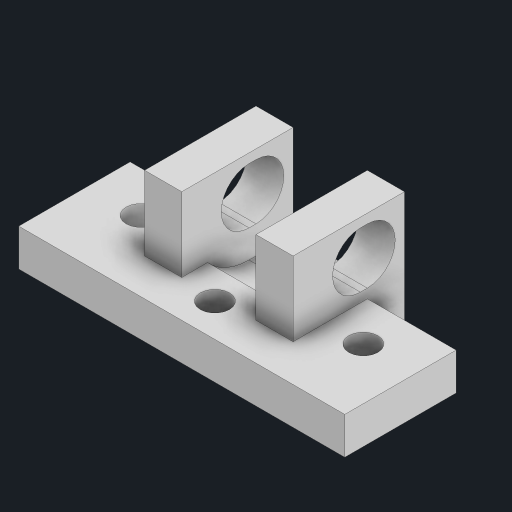
# Autodesk Inventor part: OUTK_005_LessUglyBracket
Saved by Autodesk Inventor 2024.2 (Build 282272000, 272)
## iProperties
Created: 2024-11-26
Part Number: OUTK_005_LessUglyBracket
Material: Generic
Document SubType Name: Modeling
Designer: Bryan
Density: 1 g/cm^3
Appearance: Default
Author: Bryan
Autodesk Inventor part; units mm, degrees
ref_plane "YZ Plane" through (0, 0, 0) normal (1, 0, 0) x (0, 1, 0)
ref_plane "XZ Plane" through (0, 0, 0) normal (0, 1, 0) x (-1, 0, 0)
ref_plane "XY Plane" through (0, 0, 0) normal (0, 0, 1) x (1, 0, 0)
sketch "Sketch1" plane through (0, 0, 0) normal (0, 1, 0) x (-1, 0, 0)
  circle A0 centre (0, 0) radius 2.4892
  circle A1 centre (19.05, -6.35) radius 2.4892
  circle A2 centre (-19.05, -6.35) radius 2.4892
  line L0 (21.5392, 2.4892) -> (-21.5392, 2.4892) construction
  line L1 (-21.5392, 2.4892) -> (-21.5392, -8.8392) construction
  line L2 (-21.5392, -8.8392) -> (21.5392, -8.8392) construction
  line L3 (21.5392, -8.8392) -> (21.5392, 2.4892) construction
  line L4 (27.8892, 5.6642) -> (-27.8892, 5.6642)
  line L5 (-27.8892, 5.6642) -> (-27.8892, -13.3858)
  line L6 (-27.8892, -13.3858) -> (27.8892, -13.3858)
  line L7 (27.8892, -13.3858) -> (27.8892, 5.6642)
  line L8 (12.7, -13.3858) -> (-12.7, -13.3858)
  line L9 (-12.7, -13.3858) -> (-12.7, -19.7358)
  line L10 (-12.7, -19.7358) -> (12.7, -19.7358)
  line L11 (12.7, -19.7358) -> (12.7, -13.3858)
  point P0 (21.5392, -3.175)
  point P1 (0, -19.7358)
  dimension "d0" = 4.9784
  dimension "d1" = 6.35
  dimension "d2" = 19.05
  dimension "d3" = 19.05
  dimension "d4" = 19.05
  dimension "d5" = 3.175
  dimension "d6" = 6.35
  dimension "d7" = 6.35
  dimension "d8" = 6.35
  dimension "d9" = 25.4
  constraints: 24 end point, 6 parallel, 4 tangent, 3 centre point, 3 horizontal, 3 perpendicular, 2 equal radius, 2 midpoint, 1 coincident, 1 horizontal alignment, 1 point on line, 1 vertical alignment
  measures "d0" diameter of A0
  measures "d1" vertical distance of A1.centre point (0, 0)
  measures "d2" horizontal distance of point (0, 0) A1.centre
  measures "d3" horizontal distance of A2.centre point (0, 0)
  measures "d4" distance of L5.end L4.end
  measures "d5" distance between parallel lines of L0 L4
  measures "d6" distance from line of point (21.539, -3.175) L7
  measures "d7" distance between parallel lines of L5 L1
  measures "d8" distance of L9.end L8.end
  measures "d9" distance of L9.end L10.end
extrude "Extrusion1" add sketch "Sketch1" along normal blind 6.35
sketch "Sketch2" plane through (0, 6.35, 0) normal (0, 1, 0) x (1, 0, 0)
  line L0 (-12.7, 19.7358) -> (-6.35, 19.7358)
  line L1 (-6.35, 19.7358) -> (-6.35, 0.6858)
  line L2 (-6.35, 0.6858) -> (-12.7, 0.6858)
  line L3 (-12.7, 0.6858) -> (-12.7, 19.7358)
  line L4 (12.7, 19.7358) -> (6.35, 19.7358)
  line L5 (6.35, 19.7358) -> (6.35, 0.6858)
  line L6 (6.35, 0.6858) -> (12.7, 0.6858)
  line L7 (12.7, 0.6858) -> (12.7, 19.7358)
  point P0 (0, 0)
  dimension "d12" = 6.35
  dimension "d13" = 19.05
  dimension "d14" = 6.35
  dimension "d15" = 19.05
  constraints: 16 end point, 4 parallel, 2 horizontal, 2 perpendicular, 1 coincident, 1 point on line
  measures "d12" distance of L1.end L2.end
  measures "d13" distance of L0.end L1.end
  measures "d14" distance of L6.end L5.end
  measures "d15" distance of L5.end L4.end
extrude "Extrusion2" add sketch "Sketch2" along normal blind 12.7
sketch "Sketch3" plane through (-6.35, 6.35, -0.6858) normal (1, 0, 0) x (0, 0, -1)
  circle A0 centre (12.7, 6.35) radius 9.525
  circle A1 centre (12.7, 6.35) radius 4.7625
  line L0 (0, 12.7) -> (19.05, 12.7) projected
  line L1 (19.05, -6.35) -> (19.05, 12.7) projected
  line L2 (12.7, 11.1125) -> (11.5094, 11.1125)
  circle A2 centre (11.5094, 6.35) radius 4.7625
  circle A3 centre (11.5094, 6.35) radius 9.525
  line L3 (11.5094, -3.175) -> (12.7, -3.175)
  line L4 (12.7, -3.175) -> (19.05, -3.175)
  line L5 (11.5094, 1.5875) -> (12.7, 1.5875)
  point P0 (-0.6858, -6.35)
  point P1 (19.05, -0.7495)
  point P2 (5.6005, 12.7)
  point P3 (4.4099, 12.7)
  dimension "d18" = 19.05
  dimension "d19" = 9.525
  dimension "d20" = 6.35
  dimension "d21" = 6.35
  dimension "d22" = 1.1906
  constraints: 8 end point, 4 horizontal, 4 point on circle, 3 tangent, 2 centre point, 2 coincident, 2 point on line, 1 equal radius, 6 other
  measures "d19" diameter of A1
  measures "d20" distance from line of L0 point (12.7, 6.35)
  measures "d21" distance from line of L1 point (12.7, 6.35)
  measures "d22" distance of point (12.7, 6.35) A2.centre
extrude "Extrusion3" cut sketch "Sketch3" along normal up to surface (12.7 mm away) contours A0 L1 A3 L0 | A3 L0 A0 | L1 L4 A0 | A0 A3 L1 | L0 A3 L1 A0 | A0 A3 L0 | L0 L1 A3 | L3 A3 A0 | L1 A3 | A1 A2 | A1 A2 L2 | L5 A2 A1 | A2 A1 | A1 A2 picked at (10.3907, 13.1177) picked at (2.9468, 4.8659)
extrude "Extrusion4" cut sketch "Sketch3" along normal through all both and the other way through all contours A1 A2 | A1 A2 L2 | L5 A2 A1 | A2 A1 | A1 A2
body "Solid1"
